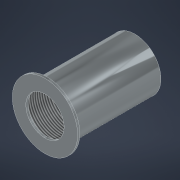
# Autodesk Inventor part: bearingShellOuter
Saved by Autodesk Inventor 2021.4 (Build 254397000, 397)
## iProperties
Created: 2022-03-02
Part Number: bearingShellOuter
Material: Generic
Document SubType Name: Modeling
Designer: jo_ki
Density: 1 g/cm^3
Appearance: Zinc
Author: jo_ki
Autodesk Inventor part; units mm, degrees
ref_plane "YZ Plane" through (0, 0, 0) normal (1, 0, 0) x (0, 1, 0)
ref_plane "XZ Plane" through (0, 0, 0) normal (0, 1, 0) x (-1, 0, 0)
ref_plane "XY Plane" through (0, 0, 0) normal (0, 0, 1) x (1, 0, 0)
sketch "Sketch2" plane through (0, 0, 0) normal (1, 0, 0) x (0, 1, 0)
  line L0 (11.5, -39) -> (10.5, -39)
  line L1 (10.5, -39) -> (10.5, 0)
  line L2 (10.5, 0) -> (11.5, 0)
  line L3 (11.5, 0) -> (11.5, -39)
  line L4 (14.5, 1) -> (8.5, 1)
  line L5 (8.5, 1) -> (8.5, 0)
  line L6 (8.5, 0) -> (14.5, 0)
  line L7 (14.5, 0) -> (14.5, 1)
  line L8 (-2.9, 0) -> (17.4, 0) projected
  line L9 (0, -47) -> (0, 9) projected
  point P0 (0, 0)
  point P1 (10.5, 0)
  dimension "d0" = 1
  dimension "d2" = 11.5
  dimension "d3" = 3
  dimension "d4" = 2
  dimension "d5" = 39
  constraints: 16 end point, 4 parallel, 3 perpendicular, 2 horizontal, 1 collinear, 1 point on line
  measures "d0" distance between parallel lines of L1 L3
  measures "d2" distance between parallel lines of L9 L3
  measures "d3" distance between parallel lines of L7 L3
  measures "d4" distance between parallel lines of L5 L1
  measures "d5" distance between parallel lines of L2 L0
revolve "Revolution1" add sketch "Sketch2" angle 360 about axis through (0, 0, -10) along (0, 0, 1)
thread "Thread1" size "M22x1" class "6H" standard "ISO Metric profile" full length
body "Solid1"
